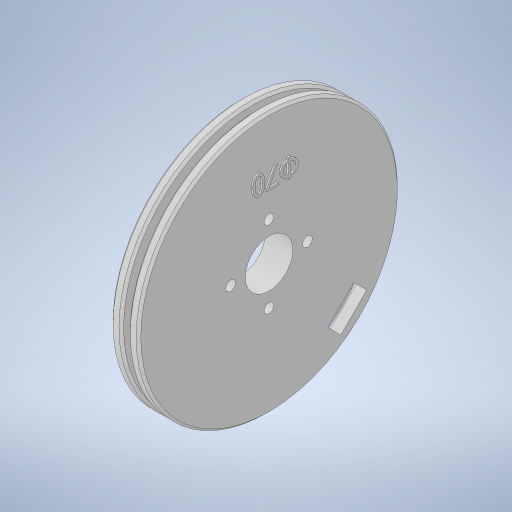
# Autodesk Inventor part: pully_shoulder2_70
Saved by Autodesk Inventor 2024 (Build 280153000, 153)
## iProperties
Created: 2025-06-10
Part Number: pully_shoulder2_70
Material: 一般
Document SubType Name: Modeling
Designer: HosodaLab2
Density: 1 g/cm^3
Appearance: 既定
Author: HosodaLab2
Autodesk Inventor part; units mm, degrees
ref_plane "YZ Plane" through (0, 0, 0) normal (1, 0, 0) x (0, 1, 0)
ref_plane "XZ Plane" through (0, 0, 0) normal (0, 1, 0) x (-1, 0, 0)
ref_plane "XY Plane" through (0, 0, 0) normal (0, 0, 1) x (1, 0, 0)
sketch "スケッチ1" plane through (0, 0, 0) normal (0, 1, 0) x (-1, 0, 0)
  circle A0 centre (0, 0) radius 35
  dimension "d0" = 70
  constraints: 1 centre point, 1 coincident
  measures "d0" diameter of A0
extrude "押し出し1" add sketch "スケッチ1" along normal blind 2.2
sketch "スケッチ2" plane through (0, 2.2, 0) normal (0, 1, 0) x (1, 0, 0)
  circle A0 centre (0, 0) radius 42.5
  line L0 (-3.2969, -22.0057) -> (4.4145, -22.0057) construction
  line L1 (4.4145, -22.0057) -> (4.4145, -25.1797) construction
  line L2 (4.4145, -25.1797) -> (-3.2969, -25.1797) construction
  line L3 (-3.2969, -25.1797) -> (-3.2969, -22.0057) construction
  dimension "d3" = 85
  constraints: 1 centre point, 1 coincident, 2 other
  measures "d3" diameter of A0
extrude "押し出し2" add sketch "スケッチ2" along normal blind 3.4
chamfer "面取り1" distance 0.75 angle 45 1 edges at (-42.5, 2.2, 0)
chamfer "面取り2" distance 0.75 angle 45 1 edges at (-42.5, 5.6, 0)
sketch "スケッチ3" plane through (0, 0, 0) normal (0, -1, 0) x (1, 0, 0)
  circle A0 centre (0, 0) radius 42.5
  dimension "d12" = 85
  constraints: 1 centre point, 1 coincident
  measures "d12" diameter of A0
extrude "押し出し3" add sketch "スケッチ3" along normal blind 3.4
chamfer "面取り3" distance 0.75 angle 45 1 edges at (-42.5, 0, 0)
chamfer "面取り4" distance 0.75 angle 45 1 edges at (-42.5, -3.4, 0)
sketch "スケッチ6" plane through (0, 5.6, 0) normal (0, 1, 0) x (1, 0, 0)
  circle A0 centre (0, 0) radius 7.65
  line L0 (0, 7.65) -> (46.8799, 7.65)
  circle A1 centre (0, 0) radius 47.5 projected
  line L1 (0, -7.65) -> (46.8799, -7.65)
  dimension "d39" = 15.3
  constraints: 4 end point, 4 point on circle, 1 centre point, 1 coincident, 1 horizontal, 1 parallel, 1 tangent
  measures "d39" diameter of A0
extrude "押し出し5" [suppressed]
chamfer "面取り7" [suppressed]
chamfer "面取り8" [suppressed]
chamfer "面取り9" [suppressed]
sketch "スケッチ7" plane through (0, 5.6, 0) normal (0, 1, 0) x (1, 0, 0)
  line L0 (-9.3358, -20.9354) -> (21.308, -20.9354) construction
  line L1 (21.308, -20.9354) -> (21.308, -27.5341) construction
  line L2 (21.308, -27.5341) -> (-9.3358, -27.5341) construction
  line L3 (-9.3358, -27.5341) -> (-9.3358, -20.9354) construction
  spline S0 degree 2 poles (-5.7914, -21.6571) (-5.2131, -21.667) (-4.2541, -22.0526) (-3.9377, -22.3739) knots 0 0 0 1 2 2 2
  spline S1 degree 2 poles (-3.9377, -22.3739) (-3.646, -22.6754) (-3.3247, -23.5207) (-3.3247, -24.0645) knots 0 0 0 1 2 2 2
  spline S2 degree 2 poles (-3.3247, -24.0645) (-3.3247, -24.633) (-3.6708, -25.5079) (-3.9772, -25.8045) knots 0 0 0 1 2 2 2
  spline S3 degree 2 poles (-3.9772, -25.8045) (-4.3084, -26.1308) (-5.2773, -26.4916) (-5.7914, -26.5015) knots 0 0 0 1 2 2 2
  line L4 (-5.7914, -26.5015) -> (-5.7914, -27.2084)
  line L5 (-5.7914, -27.2084) -> (-6.6021, -27.2084)
  line L6 (-6.6021, -27.2084) -> (-6.6021, -26.5015)
  spline S4 degree 2 poles (-6.6021, -26.5015) (-7.1162, -26.4867) (-8.0802, -26.1506) (-8.4213, -25.8144) knots 0 0 0 1 2 2 2
  spline S5 degree 2 poles (-8.4213, -25.8144) (-8.7277, -25.5129) (-9.0688, -24.628) (-9.0688, -24.0645) knots 0 0 0 1 2 2 2
  spline S6 degree 2 poles (-9.0688, -24.0645) (-9.0688, -23.5306) (-8.7426, -22.6853) (-8.446, -22.3788) knots 0 0 0 1 2 2 2
  spline S7 degree 2 poles (-8.446, -22.3788) (-8.1296, -22.0526) (-7.1805, -21.672) (-6.6021, -21.6571) knots 0 0 0 1 2 2 2
  line L7 (-6.6021, -21.6571) -> (-6.6021, -21.0096)
  line L8 (-6.6021, -21.0096) -> (-5.7914, -21.0096)
  line L9 (-5.7914, -21.0096) -> (-5.7914, -21.6571)
  spline S8 degree 2 poles (-5.7914, -25.8886) (-5.4207, -25.8787) (-4.8473, -25.6562) (-4.6594, -25.4684) knots 0 0 0 1 2 2 2
  spline S9 degree 2 poles (-4.6594, -25.4684) (-4.4073, -25.2212) (-4.17, -24.5143) (-4.17, -24.0299) knots 0 0 0 1 2 2 2
  spline S10 degree 2 poles (-4.17, -24.0299) (-4.17, -23.6245) (-4.3974, -22.9572) (-4.6248, -22.7249) knots 0 0 0 1 2 2 2
  spline S11 degree 2 poles (-4.6248, -22.7249) (-4.8374, -22.5024) (-5.4009, -22.2899) (-5.7914, -22.28) knots 0 0 0 1 2 2 2
  line L10 (-5.7914, -22.28) -> (-5.7914, -25.8886)
  spline S12 degree 2 poles (-6.6021, -22.28) (-6.9926, -22.2849) (-7.5562, -22.5074) (-7.7687, -22.7249) knots 0 0 0 1 2 2 2
  spline S13 degree 2 poles (-7.7687, -22.7249) (-7.9961, -22.9523) (-8.2235, -23.6344) (-8.2235, -24.0299) knots 0 0 0 1 2 2 2
  spline S14 degree 2 poles (-8.2235, -24.0299) (-8.2235, -24.5143) (-7.9862, -25.2262) (-7.7341, -25.4684) knots 0 0 0 1 2 2 2
  spline S15 degree 2 poles (-7.7341, -25.4684) (-7.5463, -25.6463) (-6.9729, -25.8836) (-6.6021, -25.8886) knots 0 0 0 1 2 2 2
  line L11 (-6.6021, -25.8886) -> (-6.6021, -22.28)
  line L12 (1.2181, -21.9735) -> (-1.4216, -27.159)
  line L13 (-1.4216, -27.159) -> (-2.2916, -27.159)
  line L14 (-2.2916, -27.159) -> (0.4964, -21.7758)
  line L15 (0.4964, -21.7758) -> (-2.6525, -21.7758)
  line L16 (-2.6525, -21.7758) -> (-2.6525, -21.059)
  line L17 (-2.6525, -21.059) -> (1.2181, -21.059)
  line L18 (1.2181, -21.059) -> (1.2181, -21.9735)
  spline S16 degree 2 poles (5.761, -24.109) (5.761, -25.7502) (4.8069, -27.2875) (3.8134, -27.2875) knots 0 0 0 1 2 2 2
  spline S17 degree 2 poles (3.8134, -27.2875) (2.8049, -27.2875) (1.8608, -25.7205) (1.8608, -24.1139) knots 0 0 0 1 2 2 2
  spline S18 degree 2 poles (1.8608, -24.1139) (1.8608, -22.4629) (2.8148, -20.9354) (3.8134, -20.9354) knots 0 0 0 1 2 2 2
  spline S19 degree 2 poles (3.8134, -20.9354) (4.8168, -20.9354) (5.761, -22.5173) (5.761, -24.109) knots 0 0 0 1 2 2 2
  spline S20 degree 2 poles (4.713, -25.9677) (4.8317, -25.6661) (4.9305, -24.7368) (4.9305, -24.109) knots 0 0 0 1 2 2 2
  spline S21 degree 2 poles (4.9305, -24.109) (4.9305, -23.4812) (4.8317, -22.5568) (4.7081, -22.2454) knots 0 0 0 1 2 2 2
  spline S22 degree 2 poles (4.7081, -22.2454) (4.5845, -21.9339) (4.1544, -21.6126) (3.8134, -21.6126) knots 0 0 0 1 2 2 2
  spline S23 degree 2 poles (3.8134, -21.6126) (3.4723, -21.6126) (3.0323, -21.9339) (2.9038, -22.2553) knots 0 0 0 1 2 2 2
  spline S24 degree 2 poles (2.9038, -22.2553) (2.7802, -22.5667) (2.6912, -23.5158) (2.6912, -24.1139) knots 0 0 0 1 2 2 2
  spline S25 degree 2 poles (2.6912, -24.1139) (2.6912, -24.7566) (2.7703, -25.6167) (2.8988, -25.9528) knots 0 0 0 1 2 2 2
  spline S26 degree 2 poles (2.8988, -25.9528) (3.0175, -26.2692) (3.4574, -26.6103) (3.8134, -26.6103) knots 0 0 0 1 2 2 2
  spline S27 degree 2 poles (3.8134, -26.6103) (4.1495, -26.6103) (4.5894, -26.289) (4.713, -25.9677) knots 0 0 0 1 2 2 2
  point P0 (0, 0)
  constraints: 2 other
extrude "押し出し6" add sketch "スケッチ7" along normal blind 0.5
sketch "スケッチ8" plane through (0, 5.6, 0) normal (0, 1, 0) x (1, 0, 0)
  circle A0 centre (0, 0) radius 41.75 projected
  line L0 (0, 0) -> (-30.052, 30.052) construction
  circle A1 centre (0, 0) radius 42.5 projected
  line L1 (0, 0) -> (42.5, 0) construction
  line L2 (-23.3345, 31.8198) -> (-31.8198, 23.3345)
  line L3 (-31.8198, 23.3345) -> (-27.5772, 19.0919)
  line L4 (-27.5772, 19.0919) -> (-19.0919, 27.5772)
  line L5 (-19.0919, 27.5772) -> (-23.3345, 31.8198)
  line L6 (-23.3345, 31.8198) -> (-27.5772, 19.0919) construction
  line L7 (-31.8198, 23.3345) -> (-19.0919, 27.5772) construction
  point P0 (-25.4558, 25.4558)
  dimension "d83" = 135
  dimension "d84" = 6
  dimension "d85" = 12
  dimension "d86" = 33
  constraints: 16 end point, 2 midpoint, 2 parallel, 2 perpendicular, 1 equal length, 1 horizontal, 1 point on line, 2 other
  measures "d83" angle of L1 L0
  measures "d84" distance of L3.end L2.end
  measures "d85" distance between parallel lines of L5 L3
  measures "d86" distance from line of L4 point (0, 0)
extrude "押し出し7" cut sketch "スケッチ8" against normal blind 10 contours L5 L4 L3 L2
sketch "スケッチ9" plane through (0, 5.6, 0) normal (0, 1, 0) x (1, 0, 0)
  point P0 (0, 0)
  point P1 (0, 0)
  constraints: 1 coincident
hole "穴2" at (0, 5.6, 0) direction (0, -1, 0) diameter 15.5 end through all
sketch "スケッチ10" plane through (0, 5.6, 0) normal (0, 1, 0) x (1, 0, 0)
  circle A0 centre (0, 0) radius 12.5 construction
  point P0 (0, -12.5)
  point P1 (12.5, 0)
  point P2 (0, 12.5)
  point P3 (-12.5, 0)
  dimension "d67" = 25
  dimension "d81" = 360
  constraints: 1 coincident, 1 vertical alignment, 7 other
hole "穴3" at (0, 5.6, 12.5) at (-12.5, 5.6, 0) at (0, 5.6, -12.5) at (12.5, 5.6, 0) direction (0, -1, 0) diameter 3.2 end through all
